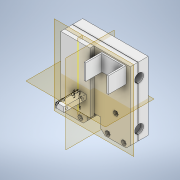
# Autodesk Inventor part: Extruder V2.1
Saved by Autodesk Inventor 2020.3 (Build 243373010, 373A)
## iProperties
Created: 2021-07-15
Part Number: Extruder V2.1
Material: ABS Plastic
Document SubType Name: Modeling
Designer: Parker
Density: 1.06 g/cm^3
Appearance: Smooth - White
Author: Parker
Autodesk Inventor part; units mm, degrees
sketch "Sketch1" plane through (0, 0, 0) normal (0, 0, 1) x (1, 0, 0)
  line L0 (-45, 45) -> (45, 45)
  line L1 (45, 45) -> (45, -45)
  line L2 (45, -45) -> (-45, -45)
  line L3 (-45, -45) -> (-45, 45)
  line L4 (-45, 45) -> (45, -45) construction
  line L5 (45, 45) -> (-45, -45) construction
  point P0 (0, 0)
  dimension "d0" = 90
  dimension "d1" = 90
  constraints: 12 end point, 2 midpoint, 2 parallel, 1 horizontal, 1 perpendicular
  measures "d0" distance of L2.end L0.start
  measures "d1" distance of L0.start L0.end
extrude "EXT Backplate Body" add sketch "Sketch1" along normal blind 5
sketch "Sketch2" plane through (0, 0, 0) normal (0, 0, -1) x (-1, 0, 0)
  line L0 (45, -45) -> (-45, -45) projected
  line L1 (45, 45) -> (45, -45) projected
  line L2 (-45, 45) -> (45, 45) projected
  line L3 (-45, -45) -> (-45, 45) projected
  point P0 (0, 0)
extrude "EXT Carriage Mount" add sketch "Sketch2" along normal blind 9.5 separate body
sketch "Sketch3" plane through (-45, -45, 0) normal (-1, 0, 0) x (0, 0, 1)
  circle A0 centre (-11, 17.5) radius 5 construction
  circle A1 centre (-11, 72.5) radius 5 construction
  line L0 (-25.6, 45) -> (10.1, 45) construction
  line L1 (0, 90) -> (0, 0) construction
  circle A2 centre (-11, 72.5) radius 9.5 construction
  circle A3 centre (-11, 17.5) radius 9.5 construction
  point P0 (0, 45)
  dimension "Rod_Diameter" = 10
  dimension "d7" = 10
  dimension "Rod_Spacing" = 55
  dimension "d9" = 27.5
  dimension "Rod_Offset" = 11
  dimension "Bearing_OD" = 19
  dimension "d12" = 19
  constraints: 4 centre point, 2 coincident, 1 vertical alignment
  measures "Rod_Diameter" diameter of A0
  measures "d7" diameter of A1
  measures "Rod_Spacing" distance of A0.centre A1.centre
  measures "d9" distance from line of L0 A0.centre
  measures "Rod_Offset" distance from line of L1 A1.centre
  measures "Bearing_OD" diameter of A2
  measures "d12" diameter of A3
ref_plane "Work Plane1" through (-12.5, 0, 0) normal (1, 0, 0) x (0, 1, 0)
sketch "Sketch5" plane through (0, 0, 0) normal (1, 0, 0) x (0, 1, 0)
  circle A0 centre (27.5, -11) radius 9.5
  point P0 (0, 0)
  dimension "d17" = 19
  constraints: 1 centre point, 1 coincident
  measures "d17" diameter of A0
extrude "CUT Carriage Mount Top Bearing Clearance" cut sketch "Sketch5" along normal mid plane 29 bodies 2
sketch "Sketch4" plane through (-45, -45, 0) normal (-1, 0, 0) x (0, 0, 1)
  circle A0 centre (-11, 72.5) radius 9.5 construction
  circle A1 centre (-11, 17.5) radius 9.5 construction
  circle A2 centre (-11, 72.5) radius 9.5
  circle A3 centre (-11, 17.5) radius 9.5
  point P0 (0, 45)
  dimension "d13" = 19
  dimension "d14" = 19
  constraints: 2 centre point, 2 coincident
  measures "d13" diameter of A2
  measures "d14" diameter of A3
hole "HOL Carriage Mount Top Rail" at (-45, 27.5, -11) direction (1, 0, 0) diameter 11 end through all bodies 2
sketch "Sketch6" plane through (-12.5, 0, 0) normal (1, 0, 0) x (0, 1, 0)
  circle A0 centre (-27.5, -11) radius 9.5
  point P0 (0, 0)
  dimension "d27" = 19
  constraints: 1 centre point, 1 coincident
  measures "d27" diameter of A0
extrude "CUT Carriage Mount Bottom Bearing Clearance" cut sketch "Sketch6" against normal blind 29 bodies 2
mirror "MIR Carriage Mount Bottom Bearings" about plane through (0, 0, 0) normal (1, 0, 0) of "CUT Carriage Mount Bottom Bearing Clearance" bodies 2
hole "HOL Carriage Mount Bottom Rail" at (-45, -27.5, -11) direction (1, 0, 0) diameter 11 end through all bodies 2
ref_plane "Work Plane3" through (0, 0, -9.9) normal (0, 0, 1) x (1, 0, 0)
sketch "Sketch7" plane through (0, 0, -9.9) normal (0, 0, 1) x (1, 0, 0)
  line L0 (45, 45) -> (-45, 45) projected
  line L1 (45, -45) -> (-45, -45)
  line L2 (-45, -45) -> (-45, 45)
  line L3 (-45, 45) -> (45, 45)
  line L4 (45, 45) -> (45, -45)
  line L5 (45, -45) -> (-45, 45) construction
  line L6 (-45, -45) -> (45, 45) construction
  point P0 (0, 0)
  dimension "d38" = 90
  dimension "d39" = 90
  constraints: 12 end point, 2 midpoint, 2 parallel, 1 horizontal, 1 perpendicular
  measures "d38" distance of L0.end L3.end
  measures "d39" distance of L1.end L0.end
extrude "Carriage Backplate Body" add sketch "Sketch7" against normal blind 12.5 separate body
sketch "Sketch8" plane through (-45, -45, -9.9) normal (-1, 0, 0) x (0, 0, 1)
  point P0 (9.9, 45)
  point P1 (-1.1, 72.5)
  point P2 (-1.1, 17.5)
hole "HOL Carriage Backplate Rail Clearance" at (-45, 27.5, -11) at (-45, -27.5, -11) direction (1, 0, 0) diameter 11 end through all bodies 3
extrude "CUT Carriage Backplate Top Bearing" cut sketch "Sketch5" against normal mid plane 29 bodies 3
extrude "CUT Carriage Backplate Bottom Bearing" cut sketch "Sketch6" against normal blind 29 bodies 3
mirror "MIR Carriage Backplate Bottom Bearings" about plane through (0, 0, 0) normal (1, 0, 0) of "CUT Carriage Backplate Bottom Bearing" bodies 3
sketch "Sketch9" plane through (0, 0, 5) normal (0, 0, 1) x (1, 0, 0)
  line L0 (-45, -45) -> (45, -45) projected
  line L1 (45, -45) -> (45, 45) projected
  line L2 (-45, -45) -> (45, -45)
  line L3 (45, -45) -> (45, -30)
  line L4 (45, -30) -> (-45, -30)
  line L5 (-45, -30) -> (-45, -45)
  point P0 (0, 0)
  dimension "d53" = 15
  constraints: 8 end point, 2 parallel, 1 horizontal, 1 perpendicular, 1 point on line
  measures "d53" distance of L3.end L2.end
extrude "Extrusion8" cut sketch "Sketch9" against normal blind 10 bodies 1
sketch "Sketch10" plane through (0, 0, -22.4) normal (0, 0, -1) x (-1, 0, 0)
  line L0 (12.5, -18.1192) -> (41.5, -18.1192) projected
  line L1 (12.5, -18.1192) -> (12.5, -36.8808) projected
  line L2 (41.5, -36.8808) -> (12.5, -36.8808) projected
  line L3 (41.5, -36.8808) -> (41.5, -18.1192) projected
  line L4 (41.5, -36.8808) -> (12.5, -36.8808) projected
  point P0 (0, 0)
  point P1 (37, -40.8808)
  point P2 (17, -40.8808)
  point P3 (27, -36.8808)
  dimension "d56" = 20
  dimension "d57" = 4
  dimension "d72" = 10
  constraints: 1 midpoint
  measures "d56" distance of point (37, -40.881) point (17, -40.881)
  measures "d57" distance from line of L2 point (17, -40.881)
  measures "d72" horizontal distance of point (27, -36.881) point (17, -40.881)
hole "Hole4" at (-37, -40.8808, -22.4) at (-17, -40.8808, -22.4) direction (0, 0, 1) diameter 3.4 end through all counterbore diameter 6.5 counterbore depth 3 bodies 3 2 clearance for "Socket Head Cap Screw" size "M3" standard "Ansi Metric M Profile"
sketch "Sketch11" plane through (0, 0, 0) normal (0, 0, 1) x (1, 0, 0)
  circle A0 centre (-37, -40.8808) radius 1.7 projected
  circle A1 centre (-17, -40.8808) radius 1.7 projected
  line L0 (-38.6166, -43.6808) -> (-40.2332, -40.8808)
  line L1 (-40.2332, -40.8808) -> (-38.6166, -38.0808)
  line L2 (-38.6166, -38.0808) -> (-35.3834, -38.0808)
  line L3 (-35.3834, -38.0808) -> (-33.7668, -40.8808)
  line L4 (-33.7668, -40.8808) -> (-35.3834, -43.6808)
  line L5 (-35.3834, -43.6808) -> (-38.6166, -43.6808)
  line L6 (-18.6166, -43.6808) -> (-20.2332, -40.8808)
  line L7 (-20.2332, -40.8808) -> (-18.6166, -38.0808)
  line L8 (-18.6166, -38.0808) -> (-15.3834, -38.0808)
  line L9 (-15.3834, -38.0808) -> (-13.7668, -40.8808)
  line L10 (-13.7668, -40.8808) -> (-15.3834, -43.6808)
  line L11 (-15.3834, -43.6808) -> (-18.6166, -43.6808)
  point P0 (0, 0)
  dimension "Nut_Trap_Width" = 5.6
  dimension "d66" = 5.6
  constraints: 24 end point, 2 coincident, 26 other
  measures "Nut_Trap_Width" distance between parallel lines of L5 L2
  measures "d66" distance between parallel lines of L11 L8
extrude "Extrusion9" cut sketch "Sketch11" against normal blind 3 contours A1 | L0 L1 L2 L3 L4 L5 | L6 L7 L8 L9 L10 L11 bodies 2
sketch "Sketch12" plane through (0, 0, -22.4) normal (0, 0, -1) x (-1, 0, 0)
  line L0 (12.5, -18.1192) -> (41.5, -18.1192) projected
  line L1 (12.5, -18.1192) -> (12.5, -36.8808) projected
  line L2 (41.5, -36.8808) -> (12.5, -36.8808) projected
  line L3 (41.5, -36.8808) -> (41.5, -18.1192) projected
  point P0 (0, 0)
  point P1 (27, -18.1192)
  point P2 (27, -14.1192)
  dimension "d73" = 4
  constraints: 1 midpoint, 1 vertical alignment
  measures "d73" distance of point (27, -18.119) point (27, -14.119)
hole "Hole5" at (-27, -14.1192, -22.4) direction (0, 0, 1) diameter 3.4 end through all counterbore diameter 6.5 counterbore depth 3 bodies 3 2 clearance for "Socket Head Cap Screw" size "M3" standard "Ansi Metric M Profile"
sketch "Sketch13" plane through (0, 0, 0) normal (0, 0, 1) x (1, 0, 0)
  circle A0 centre (-27, -14.1192) radius 1.7 projected
  line L0 (-28.6166, -16.9192) -> (-30.2332, -14.1192)
  line L1 (-30.2332, -14.1192) -> (-28.6166, -11.3192)
  line L2 (-28.6166, -11.3192) -> (-25.3834, -11.3192)
  line L3 (-25.3834, -11.3192) -> (-23.7668, -14.1192)
  line L4 (-23.7668, -14.1192) -> (-25.3834, -16.9192)
  line L5 (-25.3834, -16.9192) -> (-28.6166, -16.9192)
  point P0 (0, 0)
  dimension "d81" = 5.6
  constraints: 12 end point, 1 coincident, 13 other
  measures "d81" distance between parallel lines of L5 L2
extrude "Extrusion10" cut sketch "Sketch13" against normal blind 3 contours A0 | L0 L1 L2 L3 L4 L5 bodies 2
mirror "Mirror3" about plane through (0, 0, 0) normal (1, 0, 0) of "Hole4", "Hole5", "Extrusion9", "Extrusion10" bodies 2 3
chamfer "Chamfer2" distance 5 angle 45 4 edges at (-45, -45, -4.75) (45, -45, -4.75) (-45, -45, -16.15) (45, -45, -16.15)
sketch "Sketch14" plane through (0, 0, -22.4) normal (0, 0, -1) x (-1, 0, 0)
  line L0 (12.5, -18.1192) -> (41.5, -18.1192) projected
  line L1 (12.5, -18.1192) -> (12.5, -36.8808) projected
  line L2 (41.5, -36.8808) -> (12.5, -36.8808) projected
  line L3 (41.5, -36.8808) -> (41.5, -18.1192) projected
  line L4 (12.5, -27.5) -> (-37.9436, -27.5) construction
  line L5 (-8.5, -10) -> (8.5, -10)
  line L6 (8.5, -10) -> (8.5, -45)
  line L7 (8.5, -45) -> (-8.5, -45)
  line L8 (-8.5, -45) -> (-8.5, -10)
  line L9 (-8.5, -10) -> (8.5, -45) construction
  line L10 (8.5, -10) -> (-8.5, -45) construction
  line L11 (0, -63) -> (0, 63) projected
  line L12 (-40, -45) -> (40, -45) projected
  line L13 (8.5, -27.5) -> (-8.5, -27.5)
  point P0 (0, 0)
  point P1 (0, -27.5)
  point P2 (0, -27.5)
  point P3 (0, -45)
  dimension "d87" = 4
  constraints: 16 end point, 8 midpoint, 2 horizontal, 2 parallel, 2 point on line, 1 perpendicular
  measures "d87" distance between parallel lines of L1 L6
extrude "Extrusion11" cut sketch "Sketch14" against normal through all contours L13 L11 L7 L8 | L13 L6 L7 L11 bodies 3 2
chamfer "Chamfer3" distance 5 angle 45 4 edges at (8.5, -45, -4.75) (-8.5, -45, -4.75) (8.5, -45, -16.15) (-8.5, -45, -16.15)
sketch "Sketch15" plane through (0, 0, 5) normal (0, 0, 1) x (1, 0, 0)
  line L0 (45, -30) -> (45, 45) projected
  line L1 (-45, -30) -> (45, -30) projected
  line L2 (45, 45) -> (0, 45)
  line L3 (0, 45) -> (0, -30)
  line L4 (0, -30) -> (45, -30)
  line L5 (45, -30) -> (45, 45)
  point P0 (0, 0)
  constraints: 8 end point, 2 parallel, 1 horizontal, 1 midpoint, 1 perpendicular
extrude "Extrusion12" cut sketch "Sketch15" against normal through all bodies 1
ref_plane "Work Plane4" through (-15, -30, 5) normal (1, 0, 0) x (0, 0, -1)
sketch "Sketch16" plane through (-15, -30, 5) normal (1, 0, 0) x (0, 0, -1)
  line L0 (5, 0) -> (0, 0) projected
  line L1 (0, 75) -> (0, 0) projected
  line L2 (2.4592, 23) -> (-27.5, 23)
  line L3 (-27.5, 23) -> (-27.5, 17)
  line L4 (-27.5, 17) -> (2.4592, 17)
  line L5 (2.4592, 17) -> (2.4592, 23)
  point P0 (5, 30)
  point P1 (-4.5, 20)
  point P2 (-24.5, 20)
  point P3 (0, 17)
  point P4 (0, 23)
  dimension "d96" = 20
  dimension "d97" = 4.5
  dimension "d98" = 20
  dimension "d99" = 3
  dimension "d100" = 3
  dimension "d101" = 3
  constraints: 8 end point, 2 parallel, 1 horizontal, 1 horizontal alignment, 1 perpendicular
  measures "d96" distance from line of point (-4.5, 20) L0
  measures "d97" distance from line of point (-4.5, 20) L1
  measures "d98" distance of point (-24.5, 20) point (-4.5, 20)
  measures "d99" distance from line of L3 point (-24.5, 20)
  measures "d100" distance from line of L2 point (-4.5, 20)
  measures "d101" distance from line of L4 point (-4.5, 20)
extrude "Extrusion13" add sketch "Sketch16" along normal blind 10 contours L1 L4 L3 L2 bodies 1
hole "Hole6" at (-15, -10, 9.5) at (-15, -10, 29.5) direction (1, 0, 0) diameter 2.9 end through all bodies 1 clearance for "Socket Head Cap Screw" size "M2.5" standard "Ansi Metric M Profile"
sketch "Sketch18" plane through (0, 0, 0) normal (0, 0, 1) x (1, 0, 0)
  line L0 (9.8863, 23.6583) -> (39.8863, 23.6583)
  line L1 (39.8863, 23.6583) -> (39.8863, 43.6583)
  line L2 (39.8863, 43.6583) -> (9.8863, 43.6583)
  line L3 (9.8863, 43.6583) -> (9.8863, 23.6583)
  line L4 (9.8863, 23.6583) -> (39.8863, 43.6583) construction
  line L5 (39.8863, 23.6583) -> (9.8863, 43.6583) construction
  point P0 (24.8863, 33.6583)
  dimension "d112" = 30
  dimension "d113" = 20
  constraints: 12 end point, 2 midpoint, 2 parallel, 1 horizontal, 1 perpendicular
  measures "d112" distance of L2.end L1.end
  measures "d113" distance of L1.end L0.end
extrude "Extrusion14" add sketch "Sketch18" along normal blind 2 separate body
sketch "Sketch20" plane through (0, 0, 2) normal (0, 0, 1) x (1, 0, 0)
  line L0 (39.8863, 23.6583) -> (39.8863, 43.6583) projected
  line L1 (39.8863, 43.6583) -> (9.8863, 43.6583) projected
  line L2 (9.8863, 43.6583) -> (9.8863, 23.6583) projected
  line L3 (9.8863, 23.6583) -> (39.8863, 23.6583) projected
  line L4 (39.8863, 43.6583) -> (9.8863, 43.6583) projected
  line L5 (11.7863, 23.6583) -> (37.9863, 23.6583)
  line L6 (37.9863, 23.6583) -> (37.9863, 43.6583)
  line L7 (37.9863, 43.6583) -> (11.7863, 43.6583)
  line L8 (11.7863, 43.6583) -> (11.7863, 23.6583)
  line L9 (11.7863, 23.6583) -> (37.9863, 43.6583) construction
  line L10 (37.9863, 23.6583) -> (11.7863, 43.6583) construction
  point P0 (0, 0)
  point P1 (24.8863, 33.6583)
  dimension "d119" = 26.2
  constraints: 12 end point, 2 midpoint, 2 parallel, 1 horizontal, 1 perpendicular, 1 point on line
  measures "d119" distance of L7.end L6.end
extrude "Extrusion16" add sketch "Sketch20" along normal blind 20 contours L3 L6 L1 L0 | L3 L2 L1 L8 bodies 4
equation "\"d4\" = 0.5 * Bearing_OD"
equation "\"d7\" = Rod_Diameter"
equation "\"d9\" = 0.5 * Rod_Spacing"
equation "\"d12\" = Bearing_OD"
equation "\"d17\" = Bearing_OD"
equation "\"d13\" = Bearing_OD"
equation "\"d14\" = Bearing_OD"
equation "\"d20\" = 2 * Rod_Clearance + Rod_Diameter"
equation "\"d27\" = Bearing_OD"
equation "\"d28\" = Bearing_Length"
equation "\"d30\" = 2 * Rod_Clearance + Rod_Diameter"
equation "\"d42\" = 2 * Rod_Clearance + Rod_Diameter"
equation "\"d49\" = Bearing_Length"
equation "\"d51\" = Bearing_Length"
equation "\"d66\" = Nut_Trap_Width"
equation "\"d81\" = Nut_Trap_Width"
equation "\"Bearing_Spacing\" = 25"
equation "\"d15\" = -0.5 * Bearing_Spacing"
equation "\"Rod_Clearance\" = 0.5"
equation "\"Backplate_Clamping_Clearance\" = 0.4"
equation "\"d37\" = -0.5 * Bearing_OD - Backplate_Clamping_Clearance"
equation "\"Bearing_Length\" = 29"
body "Solid4"
